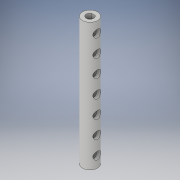
# Autodesk Inventor part: DShaftSpinner4inx12mm
Saved by Autodesk Inventor 2019 (Build 230136000, 136)
## iProperties
Created: 2018-09-29
Part Number: DShaftSpinner4inx12mm
Material: Generic
Document SubType Name: Modeling
Designer: mrhftc
Density: 1 g/cm^3
Appearance: Default
Author: mrhftc
Autodesk Inventor part; units mm, degrees
ref_plane "YZ Plane" through (0, 0, 0) normal (1, 0, 0) x (0, 1, 0)
sketch "Main Shaft Sketch" plane through (0, 0, 0) normal (0, 1, 0) x (-1, 0, 0)
  circle A0 centre (0, 0) radius 6
  line L0 (0, 7.3639) -> (0, 0)
  line L1 (0, 0) -> (0, -8.8137)
  line L2 (6.485, 0) -> (0, 0) construction
  line L3 (-6.963, 0) -> (0, 0)
  circle A1 centre (0, 0) radius 6
  arc A2 (1.6583, -2.5) -> (-1.6583, -2.5) centre (0, 0) ccw
  line L4 (1.6583, -2.5) -> (-1.6583, -2.5)
  point P0 (0, 3.0022)
  dimension "d41" = 12
  dimension "d42" = 6
  dimension "d43" = 5
  constraints: 10 end point, 3 centre point, 2 coincident, 2 horizontal, 2 point on circle, 2 point on line, 1 collinear, 1 vertical, 1 other
  measures "d41" diameter of A0
  measures "d42" diameter of A2
  measures "d43" diameter of L4 L2
ref_plane "Work Plane1" through (0, 50.8, 0) normal (0, -1, 0) x (1, 0, 0)
ref_plane "Work Plane2" through (6, 0, 0) normal (-1, 0, 0) x (0, -1, 0)
sketch "Side Holes" plane through (6, 0, 0) normal (-1, 0, 0) x (0, -1, 0)
  line L0 (-99.6, 0) -> (0, 0)
  circle A0 centre (-50.8, 0) radius 3
  circle A1 centre (-36.8, 0) radius 3
  circle A2 centre (-22.8, 0) radius 3
  circle A3 centre (-8.8, 0) radius 3
  circle A4 centre (-64.8, 0) radius 3
  circle A5 centre (-50.8, 0) radius 3
  circle A6 centre (-36.8, 0) radius 3
  circle A7 centre (-22.8, 0) radius 3
  circle A8 centre (-78.8, 0) radius 3
  circle A9 centre (-64.8, 0) radius 3
  circle A10 centre (-50.8, 0) radius 3
  circle A11 centre (-36.8, 0) radius 3
  circle A12 centre (-92.8, 0) radius 3
  circle A13 centre (-78.8, 0) radius 3
  circle A14 centre (-64.8, 0) radius 3
  circle A15 centre (-50.8, 0) radius 3
  point P0 (-1, 3.0022)
  dimension "d17" = 6
  dimension "d20" = 14
  dimension "d23" = 14
  constraints: 16 centre point, 2 end point, 2 horizontal, 1 point on line, 30 other
  measures "d17" diameter of A0
  measures "d20" distance of A0.centre A1.centre
  measures "d23" distance of A0.centre A4.centre
sketch "Inner Cut Sketch" plane through (0, 50.8, 0) normal (0, -1, 0) x (1, 0, 0)
  circle A0 centre (0, 0) radius 3.5
  dimension "d35" = 7
  constraints: 1 centre point, 1 coincident
  measures "d35" diameter of A0
extrude "Main Shaft Extrusion" add sketch "Main Shaft Sketch" along normal blind 101.6 contours A0 L1 L4 A2 L0 | L0 A2 L3 A0 | A0 L3 A2 L4 L1
extrude "Inner Cut" cut sketch "Inner Cut Sketch" along normal mid plane 94
extrude "Extrusion9" cut sketch "Side Holes" along normal through all
body "Solid2"
